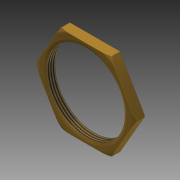
# Autodesk Inventor part: solenoid nut
Saved by Autodesk Inventor 2014 (Build 180170000, 170)
## iProperties
Created: 2013-07-22
Part Number: solenoid nut
Material: Generic
Document SubType Name: Modeling
Designer: Saville
Mass: 0.596235 g
Surface Area: 9.04193 cm^2
Volume: 0.596235 cm^3
Density: 1 g/cm^3
Appearance: Default
Author: Saville
Autodesk Inventor part; units mm, degrees
ref_plane "YZ Plane" through (0, 0, 0) normal (1, 0, 0) x (0, 1, 0)
ref_plane "XZ Plane" through (0, 0, 0) normal (0, 1, 0) x (-1, 0, 0)
ref_plane "XY Plane" through (0, 0, 0) normal (0, 0, 1) x (1, 0, 0)
sketch "Sketch1" plane through (0, 0, 0) normal (0, 0, 1) x (1, 0, 0)
  circle A0 centre (0, 0) radius 12.7 projected
  line L0 (-8.1976, -14.1986) -> (-16.3951, 0)
  line L1 (-16.3951, 0) -> (-8.1976, 14.1986)
  line L2 (-8.1976, 14.1986) -> (8.1976, 14.1986)
  line L3 (8.1976, 14.1986) -> (16.3951, 0)
  line L4 (16.3951, 0) -> (8.1976, -14.1986)
  line L5 (8.1976, -14.1986) -> (-8.1976, -14.1986)
  line L6 (-31.7325, 0) -> (27.4026, 0) construction
  line L7 (-43.5596, 0) -> (39.2297, 0) construction
  point P0 (0, 0)
  dimension "d0" = 25.4
  dimension "d1" = 28.3972
  constraints: 14 end point, 1 coincident, 1 horizontal, 1 point on line, 15 other
  measures "d0" diameter of A0
  measures "d1" distance between parallel lines of L2 L5
extrude "Extrusion1" add sketch "Sketch1" along normal blind 3.2131
thread "Thread1" size "1-32 UN" class "2B" standard "ANSI Unified Screw Threads" full length
chamfer "Chamfer1" distance 0.762 distance2 0.254 1 edges at (-12.7, 0, 3.2131) measured on face at (-0.5103, 13.6682, 3.2131)
sketch "Sketch2" plane through (0, 0, 0) normal (0, 1, 0) x (-1, 0, 0)
  line L0 (12.7, 2.9591) -> (13.462, 3.2131)
  line L1 (13.462, 3.2131) -> (16.3951, 3.2131)
  line L2 (16.3951, 3.2131) -> (16.3951, 0)
  line L3 (16.3951, 0) -> (12.7, 0)
  line L4 (12.7, 0) -> (12.7, 2.9591)
  line L5 (-12.965, 3.2131) -> (-12.7, 2.9591)
  line L6 (-12.7, 2.9591) -> (-12.7, 0)
  line L7 (-12.7, 0) -> (-16.3951, 0)
  line L8 (-16.3951, 0) -> (-16.3951, 3.2131)
  line L9 (-16.3951, 3.2131) -> (-12.965, 3.2131)
  arc A0 (-14.6801, 3.2131) -> (-16.3951, 2.6321) centre (-14.6801, 0.3912) ccw
  line L10 (0, -0.673) -> (0, 4.0377) projected
  point P0 (0, 0)
  constraints: 20 end point, 2 point on circle, 1 centre point, 1 midpoint, 1 point on line, 1 tangent
revolve "Revolution1" cut sketch "Sketch2" angle 360 about axis through (0, 0, -10) along (0, 0, 1) contours A0 L8 L9
chamfer "Chamfer2" distance 0.762 distance2 0.254 1 edges at (-12.7, 0, 0) measured on face at (-0.5103, 13.6682, 0)
fillet "Fillet1" radius 0.508 6 edges at (8.1976, 14.1986, 1.3161) (-8.1976, 14.1986, 1.3161) (-16.3951, 0, 1.3161) (-8.1976, -14.1986, 1.3161) (8.1976, -14.1986, 1.3161) (16.3951, 0, 1.3161)
fillet "Fillet2" radius 0.127 36 edges at (8.1583, 14.1305, 0) (12.2963, 7.0993, 0) (16.3165, 0, 0) (12.2963, -7.0993, 0) (8.1583, -14.1305, 0) (0, -14.1986, 0) (-8.1583, -14.1305, 0) (-12.2963, -7.0993, 0) (-16.3165, 0, 0) (-12.2963, 7.0993, 0) (-8.1583, 14.1305, 0) (0, 14.1986, 0) (0, 14.1986, 3.2131) (5.8435, 14.1986, 3.1314) (8.1583, 14.1305, 2.6901) (9.3746, 12.1599, 3.1314) (12.2963, 7.0993, 3.2131) (15.2181, 2.0387, 3.1314) (16.3165, 0, 2.6901) (15.2181, -2.0387, 3.1314) (12.2963, -7.0993, 3.2131) (9.3746, -12.1599, 3.1314) (8.1583, -14.1305, 2.6901) (5.8435, -14.1986, 3.1314) (0, -14.1986, 3.2131) (-5.8435, -14.1986, 3.1314) (-8.1583, -14.1305, 2.6901) (-9.3746, -12.1599, 3.1314) (-12.2963, -7.0993, 3.2131) (-15.2181, -2.0387, 3.1314) (-16.3165, 0, 2.6901) (-15.2181, 2.0387, 3.1314) (-12.2963, 7.0993, 3.2131) (-9.3746, 12.1599, 3.1314) (-8.1583, 14.1305, 2.6901) (-5.8435, 14.1986, 3.1314)
body "Solid1"
